Autodesk Inventor part; units mm, degrees
(part 2 of 3)
  line L955 (9.481, 12.2224) -> (9.3887, 12.173)
  line L956 (9.3887, 12.173) -> (9.2008, 12.0779)
  line L957 (9.2008, 12.0779) -> (8.8135, 11.9014)
  line L958 (8.8135, 11.9014) -> (8.4127, 11.7415)
  line L959 (8.4127, 11.7415) -> (7.9999, 11.5967)
  line L960 (7.9999, 11.5967) -> (7.5762, 11.4663)
  line L961 (7.5762, 11.4663) -> (7.1423, 11.3497)
  line L962 (7.1423, 11.3497) -> (6.777, 11.8009)
  line L963 (6.777, 11.8009) -> (6.9813, 12.201)
  line L964 (6.9813, 12.201) -> (7.1969, 12.5884)
  line L965 (7.1969, 12.5884) -> (7.4243, 12.9621)
  line L966 (7.4243, 12.9621) -> (7.6641, 13.3208)
  line L967 (7.6641, 13.3208) -> (7.9172, 13.663)
  line L968 (7.9172, 13.663) -> (8.0493, 13.827)
  line L969 (8.0493, 13.827) -> (8.1169, 13.907)
  line L970 (8.1169, 13.907) -> (8.1855, 13.9856)
  line L971 (8.1855, 13.9856) -> (7.7098, 14.6404)
  line L972 (7.7098, 14.6404) -> (7.6138, 14.5994)
  line L973 (7.6138, 14.5994) -> (7.5168, 14.5599)
  line L974 (7.5168, 14.5599) -> (7.32, 14.4849)
  line L975 (7.32, 14.4849) -> (6.9164, 14.3499)
  line L976 (6.9164, 14.3499) -> (6.5011, 14.2327)
  line L977 (6.5011, 14.2327) -> (6.0755, 14.1319)
  line L978 (6.0755, 14.1319) -> (5.6404, 14.0465)
  line L979 (5.6404, 14.0465) -> (5.1967, 13.9759)
  line L980 (5.1967, 13.9759) -> (4.8805, 14.4628)
  line L981 (4.8805, 14.4628) -> (5.1255, 14.8394)
  line L982 (5.1255, 14.8394) -> (5.3805, 15.2021)
  line L983 (5.3805, 15.2021) -> (5.6457, 15.55)
  line L984 (5.6457, 15.55) -> (5.9217, 15.8817)
  line L985 (5.9217, 15.8817) -> (6.2092, 16.1955)
  line L986 (6.2092, 16.1955) -> (6.3577, 16.3448)
  line L987 (6.3577, 16.3448) -> (6.4333, 16.4173)
  line L988 (6.4333, 16.4173) -> (6.5097, 16.4883)
  line L989 (6.5097, 16.4883) -> (6.1051, 17.1892)
  line L990 (6.1051, 17.1892) -> (6.0053, 17.1585)
  line L991 (6.0053, 17.1585) -> (5.9047, 17.1293)
  line L992 (5.9047, 17.1293) -> (5.7012, 17.0754)
  line L993 (5.7012, 17.0754) -> (5.2857, 16.9833)
  line L994 (5.2857, 16.9833) -> (4.8604, 16.9101)
  line L995 (4.8604, 16.9101) -> (4.4265, 16.8544)
  line L996 (4.4265, 16.8544) -> (3.9849, 16.8149)
  line L997 (3.9849, 16.8149) -> (3.5363, 16.7911)
  line L998 (3.5363, 16.7911) -> (3.2727, 17.3084)
  line L999 (3.2727, 17.3084) -> (3.5558, 17.6573)
  line L1000 (3.5558, 17.6573) -> (3.8472, 17.9913)
  line L1001 (3.8472, 17.9913) -> (4.1474, 18.3096)
  line L1002 (4.1474, 18.3096) -> (4.4565, 18.6106)
  line L1003 (4.4565, 18.6106) -> (4.7752, 18.8927)
  line L1004 (4.7752, 18.8927) -> (4.9385, 19.0256)
  line L1005 (4.9385, 19.0256) -> (5.0212, 19.0899)
  line L1006 (5.0212, 19.0899) -> (5.1047, 19.1525)
  line L1007 (5.1047, 19.1525) -> (4.7756, 19.8919)
  line L1008 (4.7756, 19.8919) -> (4.6731, 19.8717)
  line L1009 (4.6731, 19.8717) -> (4.5701, 19.8532)
  line L1010 (4.5701, 19.8532) -> (4.362, 19.8208)
  line L1011 (4.362, 19.8208) -> (3.9391, 19.7727)
  line L1012 (3.9391, 19.7727) -> (3.5085, 19.7444)
  line L1013 (3.5085, 19.7444) -> (3.0712, 19.7343)
  line L1014 (3.0712, 19.7343) -> (2.6279, 19.7412)
  line L1015 (2.6279, 19.7412) -> (2.1792, 19.7644)
  line L1016 (2.1792, 19.7644) -> (1.9712, 20.3064)
  line L1017 (1.9712, 20.3064) -> (2.2891, 20.6238)
  line L1018 (2.2891, 20.6238) -> (2.6139, 20.9256)
  line L1019 (2.6139, 20.9256) -> (2.9457, 21.2107)
  line L1020 (2.9457, 21.2107) -> (3.2846, 21.4778)
  line L1021 (3.2846, 21.4778) -> (3.631, 21.725)
  line L1022 (3.631, 21.725) -> (3.8074, 21.8401)
  line L1023 (3.8074, 21.8401) -> (3.8963, 21.8954)
  line L1024 (3.8963, 21.8954) -> (3.9859, 21.949)
  line L1025 (3.9859, 21.949) -> (3.7358, 22.7186)
  line L1026 (3.7358, 22.7186) -> (3.6319, 22.7093)
  line L1027 (3.6319, 22.7093) -> (3.5274, 22.7017)
  line L1028 (3.5274, 22.7017) -> (3.3171, 22.6913)
  line L1029 (3.3171, 22.6913) -> (2.8915, 22.6876)
  line L1030 (2.8915, 22.6876) -> (2.4603, 22.7045)
  line L1031 (2.4603, 22.7045) -> (2.0243, 22.7401)
  line L1032 (2.0243, 22.7401) -> (1.5842, 22.7933)
  line L1033 (1.5842, 22.7933) -> (1.1404, 22.8633)
  line L1034 (1.1404, 22.8633) -> (0.9901, 23.4241)
  line L1035 (0.9901, 23.4241) -> (1.3395, 23.7065)
  line L1036 (1.3395, 23.7065) -> (1.6941, 23.9727)
  line L1037 (1.6941, 23.9727) -> (2.0538, 24.2216)
  line L1038 (2.0538, 24.2216) -> (2.4188, 24.4518)
  line L1039 (2.4188, 24.4518) -> (2.7892, 24.6613)
  line L1040 (2.7892, 24.6613) -> (2.9766, 24.7575)
  line L1041 (2.9766, 24.7575) -> (3.0708, 24.8031)
  line L1042 (3.0708, 24.8031) -> (3.1655, 24.847)
  line L1043 (3.1655, 24.847) -> (2.9973, 25.6386)
  line L1044 (2.9973, 25.6386) -> (2.8929, 25.6402)
  line L1045 (2.8929, 25.6402) -> (2.7882, 25.6436)
  line L1046 (2.7882, 25.6436) -> (2.5779, 25.6552)
  line L1047 (2.5779, 25.6552) -> (2.1543, 25.696)
  line L1048 (2.1543, 25.696) -> (1.7273, 25.7578)
  line L1049 (1.7273, 25.7578) -> (1.2974, 25.8389)
  line L1050 (1.2974, 25.8389) -> (0.8652, 25.9378)
  line L1051 (0.8652, 25.9378) -> (0.4312, 26.0538)
  line L1052 (0.4312, 26.0538) -> (0.3404, 26.6272)
  line L1053 (0.3404, 26.6272) -> (0.7173, 26.8716)
  line L1054 (0.7173, 26.8716) -> (1.0978, 27.0992)
  line L1055 (1.0978, 27.0992) -> (1.4816, 27.3091)
  line L1056 (1.4816, 27.3091) -> (1.8686, 27.4999)
  line L1057 (1.8686, 27.4999) -> (2.2589, 27.6697)
  line L1058 (2.2589, 27.6697) -> (2.4553, 27.7456)
  line L1059 (2.4553, 27.7456) -> (2.5538, 27.7812)
  line L1060 (2.5538, 27.7812) -> (2.6526, 27.8149)
  line L1061 (2.6526, 27.8149) -> (2.568, 28.6198)
  line L1062 (2.568, 28.6198) -> (2.4644, 28.6323)
  line L1063 (2.4644, 28.6323) -> (2.3606, 28.6466)
  line L1064 (2.3606, 28.6466) -> (2.1527, 28.6801)
  line L1065 (2.1527, 28.6801) -> (1.7356, 28.765)
  line L1066 (1.7356, 28.765) -> (1.3174, 28.8711)
  line L1067 (1.3174, 28.8711) -> (0.8983, 28.9967)
  line L1068 (0.8983, 28.9967) -> (0.4789, 29.1403)
  line L1069 (0.4789, 29.1403) -> (0.0593, 29.3009)
  line L1070 (0.0593, 29.3009) -> (0.029, 29.8807)
  line L1071 (0.029, 29.8807) -> (0.4294, 30.0843)
  line L1072 (0.4294, 30.0843) -> (0.8316, 30.2709)
  line L1073 (0.8316, 30.2709) -> (1.2352, 30.4396)
  line L1074 (1.2352, 30.4396) -> (1.64, 30.5889)
  line L1075 (1.64, 30.5889) -> (2.0459, 30.7169)
  line L1076 (2.0459, 30.7169) -> (2.2492, 30.772)
  line L1077 (2.2492, 30.772) -> (2.3509, 30.797)
  line L1078 (2.3509, 30.797) -> (2.4527, 30.8203)
  line L1079 (2.4527, 30.8203) -> (2.4527, 31.6296)
  circle A0 centre (31.2249, 31.2249) radius 0.5
  line L1080 (62.4057, 32.859) -> (0.0441, 29.5908) construction
derived "Base_part.ipt"
derived "gear_central_part_30.ipt"
sketch "Sketch9" plane through (0, 0, 0) normal (0, 1, 0) x (-1, 0, 0)
  circle A0 centre (0, 0) radius 15
  arc A1 (4.5, -13.2571) -> (5.5, -12.8744) centre (0, 0) ccw
  line L0 (0, 0) -> (20.2233, 0) construction
  line L1 (0, 0) -> (0, -27.3647) construction
  line L2 (0.2121, 2.4395) -> (2.4395, 0.2121)
  line L3 (2.4395, -0.2121) -> (0.2121, -2.4395)
  line L4 (-0.2121, -2.4395) -> (-2.4395, -0.2121)
  line L5 (-2.4395, 0.2121) -> (-0.2121, 2.4395)
  line L6 (0, 2.6517) -> (0, -2.6517) construction
  line L7 (2.6517, 0) -> (-2.6517, 0) construction
  arc A2 (2.4395, -0.2121) -> (2.4395, 0.2121) centre (2.2274, 0) ccw
  arc A3 (-0.2121, -2.4395) -> (0.2121, -2.4395) centre (0, -2.2274) ccw
  arc A4 (-2.4395, 0.2121) -> (-2.4395, -0.2121) centre (-2.2274, 0) ccw
  arc A5 (0.2121, 2.4395) -> (-0.2121, 2.4395) centre (0, 2.2274) ccw
  line L8 (-3.1466, -0.9192) -> (-0.9192, -3.1466)
  arc A6 (-0.9192, -3.1466) -> (0.9192, -3.1466) centre (0, -2.2274) ccw
  line L9 (0.9192, -3.1466) -> (3.1466, -0.9192)
  arc A7 (3.1466, -0.9192) -> (3.1466, 0.9192) centre (2.2274, 0) ccw
  line L10 (3.1466, 0.9192) -> (0.9192, 3.1466)
  arc A8 (0.9192, 3.1466) -> (-0.9192, 3.1466) centre (0, 2.2274) ccw
  line L11 (-0.9192, 3.1466) -> (-3.1466, 0.9192)
  arc A9 (-3.1466, 0.9192) -> (-3.1466, -0.9192) centre (-2.2274, 0) ccw
  circle A10 centre (10, 0) radius 2.5
  arc A11 (13.4641, -0.5) -> (9.5, -3.4641) centre (10, 0) ccw
  line L12 (3.4274, -0.5) -> (6.5359, -0.5)
  line L13 (3.4274, 0.5) -> (6.5359, 0.5)
  line L14 (13.9911, 0.5) -> (13.4641, 0.5)
  line L15 (13.9911, -0.5) -> (13.4641, -0.5)
  line L16 (0, -5) -> (13.0767, -5) construction
  line L17 (0, -4.5) -> (13.2571, -4.5)
  line L18 (0, -5.5) -> (12.8744, -5.5)
  line L19 (5, 0) -> (5, -13.0767) construction
  line L20 (5.5, 12.8744) -> (5.5, -12.8744)
  line L21 (4.5, 13.2571) -> (4.5, -13.2571)
  arc A12 (0, -14) -> (4.5, -13.2571) centre (0, 0) ccw
  arc A13 (5.5, -12.8744) -> (12.8744, -5.5) centre (0, 0) ccw
  arc A14 (12.8744, -5.5) -> (13.2571, -4.5) centre (0, 0) ccw
  arc A15 (13.2571, -4.5) -> (13.9911, -0.5) centre (0, 0) ccw
  arc A16 (13.9911, -0.5) -> (13.9911, 0.5) centre (0, 0) ccw
  arc A17 (13.9911, 0.5) -> (5.5, 12.8744) centre (0, 0) ccw
  line L22 (0.5, -4.5) -> (0.5, -5.5)
  line L23 (10, 0) -> (10, -4.5) construction
  line L24 (10.5, -3.4641) -> (10.5, -4.5)
  line L25 (9.5, -3.4641) -> (9.5, -4.5)
  arc A18 (10.5, -3.4641) -> (13.4641, -0.5) centre (10, 0) ccw
  arc A19 (9.5, -3.4641) -> (10.5, -3.4641) centre (10, 0) ccw
  arc A20 (10.5, 3.4641) -> (9.5, 3.4641) centre (10, 0) ccw
  line L26 (0, -4.5) -> (0, -5.5)
  arc A21 (4.5, 13.2571) -> (0, -14) centre (0, 0) ccw
  arc A22 (5.5, 12.8744) -> (4.5, 13.2571) centre (0, 0) ccw
  line L27 (0, 4.5) -> (0, 5.5)
  line L28 (9.5, 3.4641) -> (9.5, 4.5)
  arc A23 (10.5, 3.4641) -> (9.5, 3.4641) centre (10, 0) ccw
  line L29 (0.5, 4.5) -> (0.5, 5.5)
  line L30 (0, 4.5) -> (13.2571, 4.5)
  line L31 (0, 5) -> (13.0767, 5) construction
  line L32 (0, 5.5) -> (12.8744, 5.5)
  arc A24 (13.2571, 4.5) -> (12.8744, 5.5) centre (0, 0) ccw
  line L33 (10.5, 3.4641) -> (10.5, 4.5)
  arc A25 (2.4395, -0.2121) -> (2.4395, 0.2121) centre (2.2274, 0) ccw
  line L34 (0.2121, 2.4395) -> (2.4395, 0.2121)
  line L35 (0.9192, -3.1466) -> (3.1466, -0.9192)
  arc A26 (0.2121, 2.4395) -> (-0.2121, 2.4395) centre (0, 2.2274) ccw
  line L36 (2.4395, -0.2121) -> (0.2121, -2.4395)
  line L37 (0, 2.6517) -> (0, -2.6517) construction
  line L38 (-2.4395, 0.2121) -> (-0.2121, 2.4395)
  line L39 (-2.6517, 0) -> (2.6517, 0) construction
  arc A27 (-0.2121, -2.4395) -> (0.2121, -2.4395) centre (0, -2.2274) ccw
  line L40 (-0.2121, -2.4395) -> (-2.4395, -0.2121)
  arc A28 (3.1466, -0.9192) -> (3.1466, 0.9192) centre (2.2274, 0) ccw
  line L41 (3.1466, 0.9192) -> (0.9192, 3.1466)
  line L42 (4.5, 0.5) -> (5.5, 0.5)
  line L43 (4.5, 0) -> (5.5, 0)
  line L44 (-13.2571, 4.5) -> (13.2571, 4.5)
  line L45 (0, 5) -> (13.0767, 5) construction
  arc A29 (14, 0) -> (13.2571, 4.5) centre (0, 0) ccw
  arc A30 (-0.9192, -3.1466) -> (0.9192, -3.1466) centre (0, -2.2274) ccw
  line L46 (-3.1466, -0.9192) -> (-0.9192, -3.1466)
  arc A31 (-12.8744, 5.5) -> (-13.2571, 4.5) centre (0, 0) ccw
  circle A32 centre (0, 10) radius 2.5
  arc A33 (0.5, 13.4641) -> (3.4641, 9.5) centre (0, 10) ccw
  line L47 (0.5, 3.4274) -> (0.5, 6.5359)
  line L48 (-0.5, 3.4274) -> (-0.5, 6.5359)
  arc A34 (3.4641, 10.5) -> (0.5, 13.4641) centre (0, 10) ccw
  line L49 (0, 10) -> (4.5, 10) construction
  line L50 (0.5, 13.9911) -> (0.5, 13.4641)
  arc A35 (4.5, 13.2571) -> (0.5, 13.9911) centre (0, 0) ccw
  line L51 (-12.8744, 5.5) -> (12.8744, 5.5)
  arc A36 (0.5, 13.9911) -> (-0.5, 13.9911) centre (0, 0) ccw
  line L52 (-0.5, 13.9911) -> (-0.5, 13.4641)
  arc A37 (13.2571, 4.5) -> (12.8744, 5.5) centre (0, 0) ccw
  arc A38 (3.4641, 9.5) -> (3.4641, 10.5) centre (0, 10) ccw
  line L53 (3.4641, 9.5) -> (4.5, 9.5)
  line L54 (3.4641, 10.5) -> (4.5, 10.5)
  arc A39 (5.5, 12.8744) -> (4.5, 13.2571) centre (0, 0) ccw
  line L55 (4.5, 0) -> (4.5, 13.2571)
  line L56 (5, 0) -> (5, 13.0767) construction
  line L57 (5.5, 0) -> (5.5, 12.8744)
  arc A40 (12.8744, 5.5) -> (5.5, 12.8744) centre (0, 0) ccw
  line L58 (-0.9192, 3.1466) -> (-3.1466, 0.9192)
  arc A41 (-3.4641, 10.5) -> (-3.4641, 9.5) centre (0, 10) ccw
  arc A42 (-3.4641, 10.5) -> (-3.4641, 9.5) centre (0, 10) ccw
  line L59 (-3.4641, 10.5) -> (-4.5, 10.5)
  line L60 (-4.5, 0) -> (-4.5, 13.2571)
  line L61 (-5, 0) -> (-5, 13.0767) construction
  line L62 (-5.5, 0) -> (-5.5, 12.8744)
  arc A43 (-4.5, 13.2571) -> (-5.5, 12.8744) centre (0, 0) ccw
  arc A44 (-0.5, 13.9911) -> (-12.8744, 5.5) centre (0, 0) ccw
  line L63 (-3.4641, 9.5) -> (-4.5, 9.5)
  line L64 (-4.5, 0.5) -> (-5.5, 0.5)
  line L65 (-4.5, 0) -> (-5.5, 0)
  arc A45 (-2.4395, 0.2121) -> (-2.4395, -0.2121) centre (-2.2274, 0) ccw
  arc A46 (-3.1466, 0.9192) -> (-3.1466, -0.9192) centre (-2.2274, 0) ccw
  arc A47 (0.9192, 3.1466) -> (-0.9192, 3.1466) centre (0, 2.2274) ccw
  arc A48 (0.2121, 2.4395) -> (-0.2121, 2.4395) centre (0, 2.2274) ccw
  line L66 (-2.4395, 0.2121) -> (-0.2121, 2.4395)
  line L67 (3.1466, 0.9192) -> (0.9192, 3.1466)
  arc A49 (-2.4395, 0.2121) -> (-2.4395, -0.2121) centre (-2.2274, 0) ccw
  line L68 (0.2121, 2.4395) -> (2.4395, 0.2121)
  line L69 (-2.6517, 0) -> (2.6517, 0) construction
  line L70 (-0.2121, -2.4395) -> (-2.4395, -0.2121)
  line L71 (0, -2.6517) -> (0, 2.6517) construction
  arc A50 (2.4395, -0.2121) -> (2.4395, 0.2121) centre (2.2274, 0) ccw
  line L72 (2.4395, -0.2121) -> (0.2121, -2.4395)
  arc A51 (0.9192, 3.1466) -> (-0.9192, 3.1466) centre (0, 2.2274) ccw
  line L73 (-0.9192, 3.1466) -> (-3.1466, 0.9192)
  line L74 (-0.5, 4.5) -> (-0.5, 5.5)
  line L75 (0, 4.5) -> (0, 5.5)
  line L76 (-4.5, -13.2571) -> (-4.5, 13.2571)
  line L77 (-5, 0) -> (-5, 13.0767) construction
  arc A52 (0, 14) -> (-4.5, 13.2571) centre (0, 0) ccw
  arc A53 (3.1466, -0.9192) -> (3.1466, 0.9192) centre (2.2274, 0) ccw
  line L78 (0.9192, -3.1466) -> (3.1466, -0.9192)
  arc A54 (-5.5, -12.8744) -> (-4.5, -13.2571) centre (0, 0) ccw
  circle A55 centre (-10, 0) radius 2.5
  arc A56 (-13.4641, 0.5) -> (-9.5, 3.4641) centre (-10, 0) ccw
  line L79 (-3.4274, 0.5) -> (-6.5359, 0.5)
  line L80 (-3.4274, -0.5) -> (-6.5359, -0.5)
  arc A57 (-10.5, 3.4641) -> (-13.4641, 0.5) centre (-10, 0) ccw
  line L81 (-10, 0) -> (-10, 4.5) construction
  line L82 (-13.9911, 0.5) -> (-13.4641, 0.5)
  arc A58 (-13.2571, 4.5) -> (-13.9911, 0.5) centre (0, 0) ccw
  line L83 (-5.5, -12.8744) -> (-5.5, 12.8744)
  arc A59 (-13.9911, 0.5) -> (-13.9911, -0.5) centre (0, 0) ccw
  line L84 (-13.9911, -0.5) -> (-13.4641, -0.5)
  arc A60 (-4.5, 13.2571) -> (-5.5, 12.8744) centre (0, 0) ccw
  arc A61 (-9.5, 3.4641) -> (-10.5, 3.4641) centre (-10, 0) ccw
  line L85 (-9.5, 3.4641) -> (-9.5, 4.5)
  line L86 (-10.5, 3.4641) -> (-10.5, 4.5)
  arc A62 (-12.8744, 5.5) -> (-13.2571, 4.5) centre (0, 0) ccw
  line L87 (0, 4.5) -> (-13.2571, 4.5)
  line L88 (0, 5) -> (-13.0767, 5) construction
  line L89 (0, 5.5) -> (-12.8744, 5.5)
  arc A63 (-5.5, 12.8744) -> (-12.8744, 5.5) centre (0, 0) ccw
  line L90 (-3.1466, -0.9192) -> (-0.9192, -3.1466)
  arc A64 (-10.5, -3.4641) -> (-9.5, -3.4641) centre (-10, 0) ccw
  arc A65 (-10.5, -3.4641) -> (-9.5, -3.4641) centre (-10, 0) ccw
  line L91 (-10.5, -3.4641) -> (-10.5, -4.5)
  line L92 (0, -4.5) -> (-13.2571, -4.5)
  line L93 (0, -5) -> (-13.0767, -5) construction
  line L94 (0, -5.5) -> (-12.8744, -5.5)
  arc A66 (-13.2571, -4.5) -> (-12.8744, -5.5) centre (0, 0) ccw
  arc A67 (-13.9911, -0.5) -> (-5.5, -12.8744) centre (0, 0) ccw
  line L95 (-9.5, -3.4641) -> (-9.5, -4.5)
  line L96 (-0.5, -4.5) -> (-0.5, -5.5)
  line L97 (0, -4.5) -> (0, -5.5)
  arc A68 (-0.2121, -2.4395) -> (0.2121, -2.4395) centre (0, -2.2274) ccw
  arc A69 (-0.9192, -3.1466) -> (0.9192, -3.1466) centre (0, -2.2274) ccw
  arc A70 (-3.1466, 0.9192) -> (-3.1466, -0.9192) centre (-2.2274, 0) ccw
  arc A71 (-2.4395, 0.2121) -> (-2.4395, -0.2121) centre (-2.2274, 0) ccw
  line L98 (-0.2121, -2.4395) -> (-2.4395, -0.2121)
  line L99 (-0.9192, 3.1466) -> (-3.1466, 0.9192)
  arc A72 (-0.2121, -2.4395) -> (0.2121, -2.4395) centre (0, -2.2274) ccw
  line L100 (-2.4395, 0.2121) -> (-0.2121, 2.4395)
  line L101 (0, -2.6517) -> (0, 2.6517) construction
  line L102 (2.4395, -0.2121) -> (0.2121, -2.4395)
  line L103 (2.6517, 0) -> (-2.6517, 0) construction
  arc A73 (0.2121, 2.4395) -> (-0.2121, 2.4395) centre (0, 2.2274) ccw
  line L104 (0.2121, 2.4395) -> (2.4395, 0.2121)
  arc A74 (-3.1466, 0.9192) -> (-3.1466, -0.9192) centre (-2.2274, 0) ccw
  line L105 (-3.1466, -0.9192) -> (-0.9192, -3.1466)
  line L106 (-4.5, -0.5) -> (-5.5, -0.5)
  line L107 (-4.5, 0) -> (-5.5, 0)
  line L108 (13.2571, -4.5) -> (-13.2571, -4.5)
  line L109 (0, -5) -> (-13.0767, -5) construction
  arc A75 (-14, 0) -> (-13.2571, -4.5) centre (0, 0) ccw
  arc A76 (0.9192, 3.1466) -> (-0.9192, 3.1466) centre (0, 2.2274) ccw
  line L110 (3.1466, 0.9192) -> (0.9192, 3.1466)
  arc A77 (12.8744, -5.5) -> (13.2571, -4.5) centre (0, 0) ccw
  circle A78 centre (0, -10) radius 2.5
  arc A79 (-0.5, -13.4641) -> (-3.4641, -9.5) centre (0, -10) ccw
  line L111 (-0.5, -3.4274) -> (-0.5, -6.5359)
  line L112 (0.5, -3.4274) -> (0.5, -6.5359)
  arc A80 (-3.4641, -10.5) -> (-0.5, -13.4641) centre (0, -10) ccw
  line L113 (0, -10) -> (-4.5, -10) construction
  line L114 (-0.5, -13.9911) -> (-0.5, -13.4641)
  arc A81 (-4.5, -13.2571) -> (-0.5, -13.9911) centre (0, 0) ccw
  line L115 (12.8744, -5.5) -> (-12.8744, -5.5)
  arc A82 (-0.5, -13.9911) -> (0.5, -13.9911) centre (0, 0) ccw
  line L116 (0.5, -13.9911) -> (0.5, -13.4641)
  arc A83 (-13.2571, -4.5) -> (-12.8744, -5.5) centre (0, 0) ccw
  arc A84 (-3.4641, -9.5) -> (-3.4641, -10.5) centre (0, -10) ccw
  line L117 (-3.4641, -9.5) -> (-4.5, -9.5)
  line L118 (-3.4641, -10.5) -> (-4.5, -10.5)
  arc A85 (-5.5, -12.8744) -> (-4.5, -13.2571) centre (0, 0) ccw
  line L119 (-4.5, 0) -> (-4.5, -13.2571)
  line L120 (-5, 0) -> (-5, -13.0767) construction
  line L121 (-5.5, 0) -> (-5.5, -12.8744)
  arc A86 (-12.8744, -5.5) -> (-5.5, -12.8744) centre (0, 0) ccw
  line L122 (0.9192, -3.1466) -> (3.1466, -0.9192)
  arc A87 (3.4641, -10.5) -> (3.4641, -9.5) centre (0, -10) ccw
  arc A88 (3.4641, -10.5) -> (3.4641, -9.5) centre (0, -10) ccw
  line L123 (3.4641, -10.5) -> (4.5, -10.5)
  line L124 (4.5, 0) -> (4.5, -13.2571)
  line L125 (5, 0) -> (5, -13.0767) construction
  line L126 (5.5, 0) -> (5.5, -12.8744)
  arc A89 (4.5, -13.2571) -> (5.5, -12.8744) centre (0, 0) ccw
  arc A90 (0.5, -13.9911) -> (12.8744, -5.5) centre (0, 0) ccw
  line L127 (3.4641, -9.5) -> (4.5, -9.5)
  line L128 (4.5, -0.5) -> (5.5, -0.5)
  line L129 (4.5, 0) -> (5.5, 0)
  arc A91 (2.4395, -0.2121) -> (2.4395, 0.2121) centre (2.2274, 0) ccw
  arc A92 (3.1466, -0.9192) -> (3.1466, 0.9192) centre (2.2274, 0) ccw
  arc A93 (-0.9192, -3.1466) -> (0.9192, -3.1466) centre (0, -2.2274) ccw
  point P0 (0, 2.2274)
  point P1 (10, 4.5)
  point P2 (-4.5, 10)
  point P3 (-2.2274, 0)
  point P4 (-10, -4.5)
  point P5 (0, -2.2274)
  point P6 (4.5, -10)
  point P7 (2.2274, 0)
sketch "Sketch7" plane through (0, 0, 0) normal (0, 1, 0) x (-1, 0, 0)
  line L0 (0.8173, 31.2129) -> (-0.8173, -31.2129) construction
  arc A0 (4.5, 27.4052) -> (-4.5, 27.4052) centre (0, 0) ccw
  line L1 (5.5, 13.9553) -> (5.5, 27.2222)
  line L2 (4.5, 14.3091) -> (4.5, 27.4052)
  line L3 (5.5, 0) -> (5.5, 12.8744) projected
  line L4 (4.5, 0) -> (4.5, 13.2571) projected
  line L5 (-4.5, 0) -> (-4.5, 13.2571) projected
  line L6 (-5.5, -12.8744) -> (-5.5, 12.8744) projected
  circle A1 centre (0, 0) radius 15 projected
  line L7 (-4.5, 14.3091) -> (-4.5, 27.4052)
  line L8 (-5.5, 13.9553) -> (-5.5, 27.2222)
  arc A2 (5.5, 27.2222) -> (4.5, 27.4052) centre (0, 0) ccw
  arc A3 (-5.5, 27.2222) -> (5.5, 27.2222) centre (0, 0) ccw
  arc A4 (-4.5, 27.4052) -> (-5.5, 27.2222) centre (0, 0) ccw
  arc A5 (5.5, 13.9553) -> (4.5, 14.3091) centre (0, 0) ccw
  arc A6 (-4.5, 14.3091) -> (-5.5, 13.9553) centre (0, 0) ccw
  arc A7 (-14.3091, -4.5) -> (-13.9553, -5.5) centre (0, 0) ccw
  arc A8 (-13.9553, 5.5) -> (-14.3091, 4.5) centre (0, 0) ccw
  line L9 (-13.9553, 5.5) -> (-27.2222, 5.5)
  line L10 (-14.3091, 4.5) -> (-27.4052, 4.5)
  arc A9 (-27.2222, 5.5) -> (-27.4052, 4.5) centre (0, 0) ccw
  line L11 (-14.3091, -4.5) -> (-27.4052, -4.5)
  line L12 (-13.9553, -5.5) -> (-27.2222, -5.5)
  arc A10 (-27.4052, -4.5) -> (-27.2222, -5.5) centre (0, 0) ccw
  arc A11 (4.5, -14.3091) -> (5.5, -13.9553) centre (0, 0) ccw
  arc A12 (-5.5, -13.9553) -> (-4.5, -14.3091) centre (0, 0) ccw
  line L13 (-5.5, -13.9553) -> (-5.5, -27.2222)
  line L14 (-4.5, -14.3091) -> (-4.5, -27.4052)
  arc A13 (-5.5, -27.2222) -> (-4.5, -27.4052) centre (0, 0) ccw
  line L15 (4.5, -14.3091) -> (4.5, -27.4052)
  line L16 (5.5, -13.9553) -> (5.5, -27.2222)
  arc A14 (4.5, -27.4052) -> (5.5, -27.2222) centre (0, 0) ccw
  arc A15 (14.3091, 4.5) -> (13.9553, 5.5) centre (0, 0) ccw
  arc A16 (13.9553, -5.5) -> (14.3091, -4.5) centre (0, 0) ccw
  line L17 (13.9553, -5.5) -> (27.2222, -5.5)
  line L18 (14.3091, -4.5) -> (27.4052, -4.5)
  arc A17 (27.2222, -5.5) -> (27.4052, -4.5) centre (0, 0) ccw
  line L19 (14.3091, 4.5) -> (27.4052, 4.5)
  line L20 (13.9553, 5.5) -> (27.2222, 5.5)
  arc A18 (27.4052, 4.5) -> (27.2222, 5.5) centre (0, 0) ccw
  arc A19 (14.7224, 8.5) -> (8.5, 14.7224) centre (0, 0) ccw
  line L21 (16.4545, 7.5) -> (21.7915, 7.5)
  line L22 (7.5, 16.4545) -> (7.5, 21.7915)
  arc A20 (23.6249, 10.2993) -> (10.2993, 23.6249) centre (0, 0) ccw
  arc A21 (21.7915, 7.5) -> (23.6249, 10.2993) centre (21.7915, 9.5) ccw
  arc A22 (14.7224, 8.5) -> (16.4545, 7.5) centre (16.4545, 9.5) ccw
  arc A23 (7.5, 16.4545) -> (8.5, 14.7224) centre (9.5, 16.4545) ccw
  arc A24 (10.2993, 23.6249) -> (7.5, 21.7915) centre (9.5, 21.7915) ccw
  arc A25 (-16.4545, 7.5) -> (-14.7224, 8.5) centre (-16.4545, 9.5) ccw
  line L23 (-16.4545, 7.5) -> (-21.7915, 7.5)
  arc A26 (-23.6249, 10.2993) -> (-21.7915, 7.5) centre (-21.7915, 9.5) ccw
  arc A27 (-8.5, 14.7224) -> (-14.7224, 8.5) centre (0, 0) ccw
  arc A28 (-10.2993, 23.6249) -> (-23.6249, 10.2993) centre (0, 0) ccw
  arc A29 (-8.5, 14.7224) -> (-7.5, 16.4545) centre (-9.5, 16.4545) ccw
  line L24 (-7.5, 16.4545) -> (-7.5, 21.7915)
  arc A30 (-7.5, 21.7915) -> (-10.2993, 23.6249) centre (-9.5, 21.7915) ccw
  arc A31 (-7.5, -16.4545) -> (-8.5, -14.7224) centre (-9.5, -16.4545) ccw
  line L25 (-7.5, -16.4545) -> (-7.5, -21.7915)
  arc A32 (-10.2993, -23.6249) -> (-7.5, -21.7915) centre (-9.5, -21.7915) ccw
  arc A33 (-14.7224, -8.5) -> (-8.5, -14.7224) centre (0, 0) ccw
  arc A34 (-23.6249, -10.2993) -> (-10.2993, -23.6249) centre (0, 0) ccw
  arc A35 (-14.7224, -8.5) -> (-16.4545, -7.5) centre (-16.4545, -9.5) ccw
  line L26 (-16.4545, -7.5) -> (-21.7915, -7.5)
  arc A36 (-21.7915, -7.5) -> (-23.6249, -10.2993) centre (-21.7915, -9.5) ccw
  arc A37 (16.4545, -7.5) -> (14.7224, -8.5) centre (16.4545, -9.5) ccw
  line L27 (16.4545, -7.5) -> (21.7915, -7.5)
  arc A38 (23.6249, -10.2993) -> (21.7915, -7.5) centre (21.7915, -9.5) ccw
  arc A39 (8.5, -14.7224) -> (14.7224, -8.5) centre (0, 0) ccw
  arc A40 (10.2993, -23.6249) -> (23.6249, -10.2993) centre (0, 0) ccw
  arc A41 (8.5, -14.7224) -> (7.5, -16.4545) centre (9.5, -16.4545) ccw
  line L28 (7.5, -16.4545) -> (7.5, -21.7915)
  arc A42 (7.5, -21.7915) -> (10.2993, -23.6249) centre (9.5, -21.7915) ccw
  line L29 (0, 0) -> (0, -11.3594) construction
  line L30 (-28.6518, 2.6609) -> (-28.7514, 2.692)
  line L31 (-28.7514, 2.692) -> (-28.8508, 2.725)
  line L32 (-28.8508, 2.725) -> (-29.0492, 2.7958)
  line L33 (-29.0492, 2.7958) -> (-29.4438, 2.9552)
  line L34 (-29.4438, 2.9552) -> (-29.8357, 3.1359)
  line L35 (-29.8357, 3.1359) -> (-30.2248, 3.3356)
  line L36 (-30.2248, 3.3356) -> (-30.6111, 3.5533)
  line L37 (-30.6111, 3.5533) -> (-30.9943, 3.7877)
  line L38 (-30.9943, 3.7877) -> (-30.9185, 4.3633)
  line L39 (-30.9185, 4.3633) -> (-30.4877, 4.4905)
  line L40 (-30.4877, 4.4905) -> (-30.0582, 4.6008)
  line L41 (-30.0582, 4.6008) -> (-29.6306, 4.693)
  line L42 (-29.6306, 4.693) -> (-29.2054, 4.7661)
  line L43 (-29.2054, 4.7661) -> (-28.7829, 4.8179)
  line L44 (-28.7829, 4.8179) -> (-28.573, 4.835)
  line L45 (-28.573, 4.835) -> (-28.4685, 4.8411)
  line L46 (-28.4685, 4.8411) -> (-28.3642, 4.8455)
  line L47 (-28.3642, 4.8455) -> (-28.2167, 5.6412)
  line L48 (-28.2167, 5.6412) -> (-28.3125, 5.6826)
  line L49 (-28.3125, 5.6826) -> (-28.408, 5.7258)
  line L50 (-28.408, 5.7258) -> (-28.5978, 5.817)
  line L51 (-28.5978, 5.817) -> (-28.9736, 6.0168)
  line L52 (-28.9736, 6.0168) -> (-29.3444, 6.2374)
  line L53 (-29.3444, 6.2374) -> (-29.7105, 6.4767)
  line L54 (-29.7105, 6.4767) -> (-30.072, 6.7335)
  line L55 (-30.072, 6.7335) -> (-30.4286, 7.0067)
  line L56 (-30.4286, 7.0067) -> (-30.2931, 7.5713)
  line L57 (-30.2931, 7.5713) -> (-29.8513, 7.6528)
  line L58 (-29.8513, 7.6528) -> (-29.4127, 7.7175)
  line L59 (-29.4127, 7.7175) -> (-28.9778, 7.7646)
  line L60 (-28.9778, 7.7646) -> (-28.5472, 7.7928)
  line L61 (-28.5472, 7.7928) -> (-28.1217, 7.8002)
  line L62 (-28.1217, 7.8002) -> (-27.9111, 7.7952)
  line L63 (-27.9111, 7.7952) -> (-27.8065, 7.7904)
  line L64 (-27.8065, 7.7904) -> (-27.7023, 7.7838)
  line L65 (-27.7023, 7.7838) -> (-27.4725, 8.5597)
  line L66 (-27.4725, 8.5597) -> (-27.5634, 8.611)
  line L67 (-27.5634, 8.611) -> (-27.6538, 8.6638)
  line L68 (-27.6538, 8.6638) -> (-27.8331, 8.7744)
  line L69 (-27.8331, 8.7744) -> (-28.1859, 9.0124)
  line L70 (-28.1859, 9.0124) -> (-28.5317, 9.2705)
  line L71 (-28.5317, 9.2705) -> (-28.8708, 9.5469)
  line L72 (-28.8708, 9.5469) -> (-29.2034, 9.84)
  line L73 (-29.2034, 9.84) -> (-29.5295, 10.149)
  line L74 (-29.5295, 10.149) -> (-29.3357, 10.6963)
  line L75 (-29.3357, 10.6963) -> (-28.8878, 10.7312)
  line L76 (-28.8878, 10.7312) -> (-28.4448, 10.7497)
  line L77 (-28.4448, 10.7497) -> (-28.0074, 10.751)
  line L78 (-28.0074, 10.751) -> (-27.5762, 10.7341)
  line L79 (-27.5762, 10.7341) -> (-27.1523, 10.697)
  line L80 (-27.1523, 10.697) -> (-26.9434, 10.67)
  line L81 (-26.9434, 10.67) -> (-26.8399, 10.6543)
  line L82 (-26.8399, 10.6543) -> (-26.7369, 10.6368)
  line L83 (-26.7369, 10.6368) -> (-26.4272, 11.3845)
  line L84 (-26.4272, 11.3845) -> (-26.5123, 11.4449)
  line L85 (-26.5123, 11.4449) -> (-26.5967, 11.507)
  line L86 (-26.5967, 11.507) -> (-26.7634, 11.6356)
  line L87 (-26.7634, 11.6356) -> (-27.0895, 11.9092)
  line L88 (-27.0895, 11.9092) -> (-27.4064, 12.2021)
  line L89 (-27.4064, 12.2021) -> (-27.7147, 12.5124)
  line L90 (-27.7147, 12.5124) -> (-28.0148, 12.8387)
  line L91 (-28.0148, 12.8387) -> (-28.3069, 13.1801)
  line L92 (-28.3069, 13.1801) -> (-28.0569, 13.7041)
  line L93 (-28.0569, 13.7041) -> (-27.6078, 13.692)
  line L94 (-27.6078, 13.692) -> (-27.1654, 13.6641)
  line L95 (-27.1654, 13.6641) -> (-26.7302, 13.6197)
  line L96 (-26.7302, 13.6197) -> (-26.3032, 13.5578)
  line L97 (-26.3032, 13.5578) -> (-25.8854, 13.4766)
  line L98 (-25.8854, 13.4766) -> (-25.6805, 13.4279)
  line L99 (-25.6805, 13.4279) -> (-25.5791, 13.4014)
  line L100 (-25.5791, 13.4014) -> (-25.4786, 13.3733)
  line L101 (-25.4786, 13.3733) -> (-25.0925, 14.0845)
  line L102 (-25.0925, 14.0845) -> (-25.1708, 14.1535)
  line L103 (-25.1708, 14.1535) -> (-25.2482, 14.2241)
  line L104 (-25.2482, 14.2241) -> (-25.4006, 14.3695)
  line L105 (-25.4006, 14.3695) -> (-25.6962, 14.6756)
  line L106 (-25.6962, 14.6756) -> (-25.9808, 15)
  line L107 (-25.9808, 15) -> (-26.255, 15.3408)
  line L108 (-26.255, 15.3408) -> (-26.5194, 15.6967)
  line L109 (-26.5194, 15.6967) -> (-26.7741, 16.0667)
  line L110 (-26.7741, 16.0667) -> (-26.4708, 16.5618)
  line L111 (-26.4708, 16.5618) -> (-26.0254, 16.5028)
  line L112 (-26.0254, 16.5028) -> (-25.5883, 16.4288)
  line L113 (-25.5883, 16.4288) -> (-25.1601, 16.3392)
  line L114 (-25.1601, 16.3392) -> (-24.7419, 16.2329)
  line L115 (-24.7419, 16.2329) -> (-24.3349, 16.1085)
  line L116 (-24.3349, 16.1085) -> (-24.1362, 16.0387)
  line L117 (-24.1362, 16.0387) -> (-24.0382, 16.0018)
  line L118 (-24.0382, 16.0018) -> (-23.9412, 15.9633)
  line L119 (-23.9412, 15.9633) -> (-23.4828, 16.6303)
  line L120 (-23.4828, 16.6303) -> (-23.5534, 16.7071)
  line L121 (-23.5534, 16.7071) -> (-23.6231, 16.7853)
  line L122 (-23.6231, 16.7853) -> (-23.7594, 16.9458)
  line L123 (-23.7594, 16.9458) -> (-24.0214, 17.2812)
  line L124 (-24.0214, 17.2812) -> (-24.2705, 17.6336)
  line L125 (-24.2705, 17.6336) -> (-24.5076, 18.0012)
  line L126 (-24.5076, 18.0012) -> (-24.7333, 18.3827)
  line L127 (-24.7333, 18.3827) -> (-24.948, 18.7774)
  line L128 (-24.948, 18.7774) -> (-24.5946, 19.238)
  line L129 (-24.5946, 19.238) -> (-24.1578, 19.1328)
  line L130 (-24.1578, 19.1328) -> (-23.7308, 19.0135)
  line L131 (-23.7308, 19.0135) -> (-23.3144, 18.8796)
  line L132 (-23.3144, 18.8796) -> (-22.9096, 18.7302)
  line L133 (-22.9096, 18.7302) -> (-22.5178, 18.5639)
  line L134 (-22.5178, 18.5639) -> (-22.3275, 18.4738)
  line L135 (-22.3275, 18.4738) -> (-22.2339, 18.4268)
  line L136 (-22.2339, 18.4268) -> (-22.1414, 18.3784)
  line L137 (-22.1414, 18.3784) -> (-21.6158, 18.9938)
  line L138 (-21.6158, 18.9938) -> (-21.6781, 19.0776)
  line L139 (-21.6781, 19.0776) -> (-21.7391, 19.1626)
  line L140 (-21.7391, 19.1626) -> (-21.8579, 19.3365)
  line L141 (-21.8579, 19.3365) -> (-22.0835, 19.6974)
  line L142 (-22.0835, 19.6974) -> (-22.2943, 20.0739)
  line L143 (-22.2943, 20.0739) -> (-22.4917, 20.4643)
  line L144 (-22.4917, 20.4643) -> (-22.6763, 20.8674)
  line L145 (-22.6763, 20.8674) -> (-22.8486, 21.2823)
  line L146 (-22.8486, 21.2823) -> (-22.4489, 21.7035)
  line L147 (-22.4489, 21.7035) -> (-22.0256, 21.5531)
  line L148 (-22.0256, 21.5531) -> (-21.6134, 21.3899)
  line L149 (-21.6134, 21.3899) -> (-21.2132, 21.2132)
  line L150 (-21.2132, 21.2132) -> (-20.8262, 21.0223)
  line L151 (-20.8262, 21.0223) -> (-20.454, 20.816)
  line L152 (-20.454, 20.816) -> (-20.2741, 20.7064)
  line L153 (-20.2741, 20.7064) -> (-20.1859, 20.6499)
  line L154 (-20.1859, 20.6499) -> (-20.099, 20.5921)
  line L155 (-20.099, 20.5921) -> (-19.512, 21.1492)
  line L156 (-19.512, 21.1492) -> (-19.5652, 21.239)
  line L157 (-19.5652, 21.239) -> (-19.617, 21.33)
  line L158 (-19.617, 21.33) -> (-19.717, 21.5154)
  line L159 (-19.717, 21.5154) -> (-19.9035, 21.8979)
  line L160 (-19.9035, 21.8979) -> (-20.0739, 22.2943)
  line L161 (-20.0739, 22.2943) -> (-20.2294, 22.7032)
  line L162 (-20.2294, 22.7032) -> (-20.3709, 23.1234)
  line L163 (-20.3709, 23.1234) -> (-20.4988, 23.5541)
  line L164 (-20.4988, 23.5541) -> (-20.0573, 23.9311)
  line L165 (-20.0573, 23.9311) -> (-19.652, 23.7374)
  line L166 (-19.652, 23.7374) -> (-19.2591, 23.5319)
  line L167 (-19.2591, 23.5319) -> (-18.8796, 23.3144)
  line L168 (-18.8796, 23.3144) -> (-18.5147, 23.0841)
  line L169 (-18.5147, 23.0841) -> (-18.1661, 22.84)
  line L170 (-18.1661, 22.84) -> (-17.9987, 22.7122)
  line L171 (-17.9987, 22.7122) -> (-17.9169, 22.6468)
  line L172 (-17.9169, 22.6468) -> (-17.8365, 22.5802)
  line L173 (-17.8365, 22.5802) -> (-17.1944, 23.0729)
  line L174 (-17.1944, 23.0729) -> (-17.2379, 23.1678)
  line L175 (-17.2379, 23.1678) -> (-17.2799, 23.2637)
  line L176 (-17.2799, 23.2637) -> (-17.36, 23.4585)
  line L177 (-17.36, 23.4585) -> (-17.5056, 23.8584)
  line L178 (-17.5056, 23.8584) -> (-17.6336, 24.2705)
  line L179 (-17.6336, 24.2705) -> (-17.7455, 24.6934)
  line L180 (-17.7455, 24.6934) -> (-17.8422, 25.1261)
  line L181 (-17.8422, 25.1261) -> (-17.9245, 25.5677)
  line L182 (-17.9245, 25.5677) -> (-17.446, 25.8966)
  line L183 (-17.446, 25.8966) -> (-17.0631, 25.6615)
  line L184 (-17.0631, 25.6615) -> (-16.6939, 25.4161)
  line L185 (-16.6939, 25.4161) -> (-16.3392, 25.1601)
  line L186 (-16.3392, 25.1601) -> (-16.0003, 24.8929)
  line L187 (-16.0003, 24.8929) -> (-15.6791, 24.6137)
  line L188 (-15.6791, 24.6137) -> (-15.526, 24.4692)
  line L189 (-15.526, 24.4692) -> (-15.4515, 24.3955)
  line L190 (-15.4515, 24.3955) -> (-15.3785, 24.3209)
  line L191 (-15.3785, 24.3209) -> (-14.6884, 24.7438)
  line L192 (-14.6884, 24.7438) -> (-14.7218, 24.8427)
  line L193 (-14.7218, 24.8427) -> (-14.7535, 24.9425)
  line L194 (-14.7535, 24.9425) -> (-14.8128, 25.1446)
  line L195 (-14.8128, 25.1446) -> (-14.9158, 25.5575)
  line L196 (-14.9158, 25.5575) -> (-15, 25.9808)
  line L197 (-15, 25.9808) -> (-15.0671, 26.413)
  line L198 (-15.0671, 26.413) -> (-15.1181, 26.8534)
  line L199 (-15.1181, 26.8534) -> (-15.1537, 27.3013)
  line L200 (-15.1537, 27.3013) -> (-14.6435, 27.5783)
  line L201 (-14.6435, 27.5783) -> (-14.2873, 27.3045)
  line L202 (-14.2873, 27.3045) -> (-13.9457, 27.0219)
  line L203 (-13.9457, 27.0219) -> (-13.6197, 26.7302)
  line L204 (-13.6197, 26.7302) -> (-13.3106, 26.4291)
  line L205 (-13.3106, 26.4291) -> (-13.0204, 26.1178)
  line L206 (-13.0204, 26.1178) -> (-12.8832, 25.958)
  line L207 (-12.8832, 25.958) -> (-12.8168, 25.877)
  line L208 (-12.8168, 25.877) -> (-12.752, 25.7952)
  line L209 (-12.752, 25.7952) -> (-12.0215, 26.1436)
  line L210 (-12.0215, 26.1436) -> (-12.0444, 26.2455)
  line L211 (-12.0444, 26.2455) -> (-12.0655, 26.348)
  line L212 (-12.0655, 26.348) -> (-12.1033, 26.5552)
  line L213 (-12.1033, 26.5552) -> (-12.1626, 26.9767)
  line L214 (-12.1626, 26.9767) -> (-12.2021, 27.4064)
  line L215 (-12.2021, 27.4064) -> (-12.2236, 27.8433)
  line L216 (-12.2236, 27.8433) -> (-12.2283, 28.2866)
  line L217 (-12.2283, 28.2866) -> (-12.2169, 28.7357)
  line L218 (-12.2169, 28.7357) -> (-11.6805, 28.9579)
  line L219 (-11.6805, 28.9579) -> (-11.3549, 28.6484)
  line L220 (-11.3549, 28.6484) -> (-11.0447, 28.3316)
  line L221 (-11.0447, 28.3316) -> (-10.751, 28.0074)
  line L222 (-10.751, 28.0074) -> (-10.4751, 27.6756)
  line L223 (-10.4751, 27.6756) -> (-10.219, 27.3357)
  line L224 (-10.219, 27.3357) -> (-10.0993, 27.1625)
  line L225 (-10.0993, 27.1625) -> (-10.0417, 27.075)
  line L226 (-10.0417, 27.075) -> (-9.9858, 26.9868)
  line L227 (-9.9858, 26.9868) -> (-9.2229, 27.257)
  line L228 (-9.2229, 27.257) -> (-9.235, 27.3607)
  line L229 (-9.235, 27.3607) -> (-9.2453, 27.4649)
  line L230 (-9.2453, 27.4649) -> (-9.2613, 27.6749)
  line L231 (-9.2613, 27.6749) -> (-9.2761, 28.1002)
  line L232 (-9.2761, 28.1002) -> (-9.2705, 28.5317)
  line L233 (-9.2705, 28.5317) -> (-9.2463, 28.9685)
  line L234 (-9.2463, 28.9685) -> (-9.2046, 29.4098)
  line L235 (-9.2046, 29.4098) -> (-9.1463, 29.8553)
  line L236 (-9.1463, 29.8553) -> (-8.5896, 30.0202)
  line L237 (-8.5896, 30.0202) -> (-8.2981, 29.6783)
  line L238 (-8.2981, 29.6783) -> (-8.0228, 29.3309)
  line L239 (-8.0228, 29.3309) -> (-7.7646, 28.9778)
  line L240 (-7.7646, 28.9778) -> (-7.5249, 28.619)
  line L241 (-7.5249, 28.619) -> (-7.3057, 28.2542)
  line L242 (-7.3057, 28.2542) -> (-7.2047, 28.0694)
  line L243 (-7.2047, 28.0694) -> (-7.1566, 27.9763)
  line L244 (-7.1566, 27.9763) -> (-7.1102, 27.8828)
  line L245 (-7.1102, 27.8828) -> (-6.3233, 28.0717)
  line L246 (-6.3233, 28.0717) -> (-6.3244, 28.1761)
  line L247 (-6.3244, 28.1761) -> (-6.3238, 28.2808)
  line L248 (-6.3238, 28.2808) -> (-6.3177, 28.4913)
  line L249 (-6.3177, 28.4913) -> (-6.288, 28.9159)
  line L250 (-6.288, 28.9159) -> (-6.2373, 29.3444)
  line L251 (-6.2373, 29.3444) -> (-6.1676, 29.7763)
  line L252 (-6.1676, 29.7763) -> (-6.08, 30.2109)
  line L253 (-6.08, 30.2109) -> (-5.9755, 30.6478)
  line L254 (-5.9755, 30.6478) -> (-5.4046, 30.7536)
  line L255 (-5.4046, 30.7536) -> (-5.1504, 30.3832)
  line L256 (-5.1504, 30.3832) -> (-4.9129, 30.0088)
  line L257 (-4.9129, 30.0088) -> (-4.693, 29.6306)
  line L258 (-4.693, 29.6306) -> (-4.4922, 29.2487)
  line L259 (-4.4922, 29.2487) -> (-4.3123, 28.863)
  line L260 (-4.3123, 28.863) -> (-4.2312, 28.6687)
  line L261 (-4.2312, 28.6687) -> (-4.1931, 28.5711)
  line L262 (-4.1931, 28.5711) -> (-4.1567, 28.4733)
  line L263 (-4.1567, 28.4733) -> (-3.3543, 28.5789)
  line L264 (-3.3543, 28.5789) -> (-3.3446, 28.6828)
  line L265 (-3.3446, 28.6828) -> (-3.333, 28.7869)
  line L266 (-3.333, 28.7869) -> (-3.305, 28.9957)
  line L267 (-3.305, 28.9957) -> (-3.231, 29.4148)
  line L268 (-3.231, 29.4148) -> (-3.1359, 29.8357)
  line L269 (-3.1359, 29.8357) -> (-3.0213, 30.2578)
  line L270 (-3.0213, 30.2578) -> (-2.8888, 30.6809)
  line L271 (-2.8888, 30.6809) -> (-2.7392, 31.1045)
  line L272 (-2.7392, 31.1045) -> (-2.1604, 31.1501)
  line L273 (-2.1604, 31.1501) -> (-1.9463, 30.7551)
  line L274 (-1.9463, 30.7551) -> (-1.7492, 30.358)
  line L275 (-1.7492, 30.358) -> (-1.5701, 29.9589)
  line L276 (-1.5701, 29.9589) -> (-1.4102, 29.5581)
  line L277 (-1.4102, 29.5581) -> (-1.2716, 29.1557)
  line L278 (-1.2716, 29.1557) -> (-1.2113, 28.9539)
  line L279 (-1.2113, 28.9539) -> (-1.1836, 28.8529)
  line L280 (-1.1836, 28.8529) -> (-1.1577, 28.7518)
  line L281 (-1.1577, 28.7518) -> (-0.3487, 28.773)
  line L282 (-0.3487, 28.773) -> (-0.3281, 28.8753)
  line L283 (-0.3281, 28.8753) -> (-0.3057, 28.9776)
  line L284 (-0.3057, 28.9776) -> (-0.256, 29.1823)
  line L285 (-0.256, 29.1823) -> (-0.1387, 29.5914)
  line L286 (-0.1387, 29.5914) -> (0, 30)
  line L287 (0, 30) -> (0.158, 30.4079)
  line L288 (0.158, 30.4079) -> (0.3341, 30.8148)
  line L289 (0.3341, 30.8148) -> (0.5271, 31.2205)
  line L290 (0.5271, 31.2205) -> (1.1075, 31.2053)
  line L291 (1.1075, 31.2053) -> (1.2791, 30.7901)
  line L292 (1.2791, 30.7901) -> (1.4336, 30.3745)
  line L293 (1.4336, 30.3745) -> (1.5701, 29.9589)
  line L294 (1.5701, 29.9589) -> (1.6872, 29.5436)
  line L295 (1.6872, 29.5436) -> (1.7829, 29.1289)
  line L296 (1.7829, 29.1289) -> (1.8218, 28.9219)
  line L297 (1.8218, 28.9219) -> (1.8388, 28.8186)
  line L298 (1.8388, 28.8186) -> (1.854, 28.7153)
  line L299 (1.854, 28.7153) -> (2.6608, 28.6518)
  line L300 (2.6608, 28.6518) -> (2.692, 28.7514)
  line L301 (2.692, 28.7514) -> (2.725, 28.8508)
  line L302 (2.725, 28.8508) -> (2.7958, 29.0492)
  line L303 (2.7958, 29.0492) -> (2.9552, 29.4438)
  line L304 (2.9552, 29.4438) -> (3.1359, 29.8357)
  line L305 (3.1359, 29.8357) -> (3.3356, 30.2248)
  line L306 (3.3356, 30.2248) -> (3.5533, 30.6111)
  line L307 (3.5533, 30.6111) -> (3.7877, 30.9943)
  line L308 (3.7877, 30.9943) -> (4.3633, 30.9185)
  line L309 (4.3633, 30.9185) -> (4.4905, 30.4877)
  line L310 (4.4905, 30.4877) -> (4.6008, 30.0582)
  line L311 (4.6008, 30.0582) -> (4.693, 29.6307)
  line L312 (4.693, 29.6307) -> (4.7661, 29.2054)
  line L313 (4.7661, 29.2054) -> (4.8179, 28.783)
  line L314 (4.8179, 28.783) -> (4.835, 28.5731)
  line L315 (4.835, 28.5731) -> (4.8411, 28.4685)
  line L316 (4.8411, 28.4685) -> (4.8454, 28.3642)
  line L317 (4.8454, 28.3642) -> (5.6412, 28.2167)
  line L318 (5.6412, 28.2167) -> (5.6826, 28.3125)
  line L319 (5.6826, 28.3125) -> (5.7258, 28.408)
  line L320 (5.7258, 28.408) -> (5.817, 28.5978)
  line L321 (5.817, 28.5978) -> (6.0168, 28.9736)
  line L322 (6.0168, 28.9736) -> (6.2373, 29.3444)
  line L323 (6.2373, 29.3444) -> (6.4767, 29.7106)
  line L324 (6.4767, 29.7106) -> (6.7335, 30.072)
  line L325 (6.7335, 30.072) -> (7.0067, 30.4286)
  line L326 (7.0067, 30.4286) -> (7.5713, 30.2931)
  line L327 (7.5713, 30.2931) -> (7.6528, 29.8513)
  line L328 (7.6528, 29.8513) -> (7.7175, 29.4127)
  line L329 (7.7175, 29.4127) -> (7.7646, 28.9778)
  line L330 (7.7646, 28.9778) -> (7.7928, 28.5472)
  line L331 (7.7928, 28.5472) -> (7.8002, 28.1217)
  line L332 (7.8002, 28.1217) -> (7.7952, 27.9111)
  line L333 (7.7952, 27.9111) -> (7.7904, 27.8065)
  line L334 (7.7904, 27.8065) -> (7.7838, 27.7023)
  line L335 (7.7838, 27.7023) -> (8.5597, 27.4725)
  line L336 (8.5597, 27.4725) -> (8.6109, 27.5634)
  line L337 (8.6109, 27.5634) -> (8.6638, 27.6538)
  line L338 (8.6638, 27.6538) -> (8.7744, 27.8331)
  line L339 (8.7744, 27.8331) -> (9.0124, 28.1859)
  line L340 (9.0124, 28.1859) -> (9.2705, 28.5317)
  line L341 (9.2705, 28.5317) -> (9.5468, 28.8708)
  line L342 (9.5468, 28.8708) -> (9.84, 29.2034)
  line L343 (9.84, 29.2034) -> (10.149, 29.5295)
  line L344 (10.149, 29.5295) -> (10.6963, 29.3357)
  line L345 (10.6963, 29.3357) -> (10.7312, 28.8878)
  line L346 (10.7312, 28.8878) -> (10.7497, 28.4449)
  line L347 (10.7497, 28.4449) -> (10.751, 28.0074)
  line L348 (10.751, 28.0074) -> (10.734, 27.5762)
  line L349 (10.734, 27.5762) -> (10.697, 27.1523)
  line L350 (10.697, 27.1523) -> (10.67, 26.9434)
  line L351 (10.67, 26.9434) -> (10.6543, 26.8398)
  line L352 (10.6543, 26.8398) -> (10.6368, 26.737)
  line L353 (10.6368, 26.737) -> (11.3845, 26.4272)
  line L354 (11.3845, 26.4272) -> (11.4449, 26.5123)
  line L355 (11.4449, 26.5123) -> (11.507, 26.5967)
  line L356 (11.507, 26.5967) -> (11.6356, 26.7635)
  line L357 (11.6356, 26.7635) -> (11.9092, 27.0895)
  line L358 (11.9092, 27.0895) -> (12.2021, 27.4064)
  line L359 (12.2021, 27.4064) -> (12.5124, 27.7147)
  line L360 (12.5124, 27.7147) -> (12.8387, 28.0148)
  line L361 (12.8387, 28.0148) -> (13.1801, 28.3069)
  line L362 (13.1801, 28.3069) -> (13.7041, 28.057)
  line L363 (13.7041, 28.057) -> (13.692, 27.6079)
  line L364 (13.692, 27.6079) -> (13.6641, 27.1654)
  line L365 (13.6641, 27.1654) -> (13.6197, 26.7302)
  line L366 (13.6197, 26.7302) -> (13.5577, 26.3032)
  line L367 (13.5577, 26.3032) -> (13.4766, 25.8854)
  line L368 (13.4766, 25.8854) -> (13.4279, 25.6805)
  line L369 (13.4279, 25.6805) -> (13.4014, 25.5791)
  line L370 (13.4014, 25.5791) -> (13.3733, 25.4786)
  line L371 (13.3733, 25.4786) -> (14.0845, 25.0925)
  line L372 (14.0845, 25.0925) -> (14.1535, 25.1708)
  line L373 (14.1535, 25.1708) -> (14.2241, 25.2482)
  line L374 (14.2241, 25.2482) -> (14.3695, 25.4006)
  line L375 (14.3695, 25.4006) -> (14.6756, 25.6962)
  line L376 (14.6756, 25.6962) -> (15, 25.9808)
  line L377 (15, 25.9808) -> (15.3408, 26.255)
  line L378 (15.3408, 26.255) -> (15.6967, 26.5194)
  line L379 (15.6967, 26.5194) -> (16.0667, 26.7741)
  line L380 (16.0667, 26.7741) -> (16.5618, 26.4708)
  line L381 (16.5618, 26.4708) -> (16.5028, 26.0254)
  line L382 (16.5028, 26.0254) -> (16.4288, 25.5883)
  line L383 (16.4288, 25.5883) -> (16.3392, 25.1601)
  line L384 (16.3392, 25.1601) -> (16.2329, 24.7419)
  line L385 (16.2329, 24.7419) -> (16.1085, 24.3349)
  line L386 (16.1085, 24.3349) -> (16.0387, 24.1362)
  line L387 (16.0387, 24.1362) -> (16.0018, 24.0382)
  line L388 (16.0018, 24.0382) -> (15.9633, 23.9412)
  line L389 (15.9633, 23.9412) -> (16.6303, 23.4828)
  line L390 (16.6303, 23.4828) -> (16.7071, 23.5535)
  line L391 (16.7071, 23.5535) -> (16.7853, 23.6231)
  line L392 (16.7853, 23.6231) -> (16.9458, 23.7594)
  line L393 (16.9458, 23.7594) -> (17.2812, 24.0214)
  line L394 (17.2812, 24.0214) -> (17.6336, 24.2705)
  line L395 (17.6336, 24.2705) -> (18.0012, 24.5076)
  line L396 (18.0012, 24.5076) -> (18.3827, 24.7333)
  line L397 (18.3827, 24.7333) -> (18.7774, 24.948)
  line L398 (18.7774, 24.948) -> (19.238, 24.5946)
  line L399 (19.238, 24.5946) -> (19.1328, 24.1578)
  line L400 (19.1328, 24.1578) -> (19.0135, 23.7308)
  line L401 (19.0135, 23.7308) -> (18.8796, 23.3144)
  line L402 (18.8796, 23.3144) -> (18.7302, 22.9096)
  line L403 (18.7302, 22.9096) -> (18.5639, 22.5178)
  line L404 (18.5639, 22.5178) -> (18.4738, 22.3275)
  line L405 (18.4738, 22.3275) -> (18.4268, 22.2339)
  line L406 (18.4268, 22.2339) -> (18.3784, 22.1414)
  line L407 (18.3784, 22.1414) -> (18.9938, 21.6158)
  line L408 (18.9938, 21.6158) -> (19.0776, 21.6781)
  line L409 (19.0776, 21.6781) -> (19.1626, 21.7391)
  line L410 (19.1626, 21.7391) -> (19.3365, 21.8579)
  line L411 (19.3365, 21.8579) -> (19.6974, 22.0835)
  line L412 (19.6974, 22.0835) -> (20.0739, 22.2943)
  line L413 (20.0739, 22.2943) -> (20.4643, 22.4917)
  line L414 (20.4643, 22.4917) -> (20.8674, 22.6763)
  line L415 (20.8674, 22.6763) -> (21.2823, 22.8486)
  line L416 (21.2823, 22.8486) -> (21.7035, 22.4489)
  line L417 (21.7035, 22.4489) -> (21.5531, 22.0256)
  line L418 (21.5531, 22.0256) -> (21.3899, 21.6134)
  line L419 (21.3899, 21.6134) -> (21.2132, 21.2132)
  line L420 (21.2132, 21.2132) -> (21.0223, 20.8262)
  line L421 (21.0223, 20.8262) -> (20.816, 20.454)
  line L422 (20.816, 20.454) -> (20.7064, 20.2741)
  line L423 (20.7064, 20.2741) -> (20.6499, 20.1859)
  line L424 (20.6499, 20.1859) -> (20.5921, 20.099)
  line L425 (20.5921, 20.099) -> (21.1492, 19.512)
  line L426 (21.1492, 19.512) -> (21.239, 19.5652)
  line L427 (21.239, 19.5652) -> (21.33, 19.617)
  line L428 (21.33, 19.617) -> (21.5154, 19.717)
  line L429 (21.5154, 19.717) -> (21.8979, 19.9035)
  line L430 (21.8979, 19.9035) -> (22.2943, 20.0739)
  line L431 (22.2943, 20.0739) -> (22.7032, 20.2294)
  line L432 (22.7032, 20.2294) -> (23.1234, 20.3709)
  line L433 (23.1234, 20.3709) -> (23.5541, 20.4988)
  line L434 (23.5541, 20.4988) -> (23.9311, 20.0573)
  line L435 (23.9311, 20.0573) -> (23.7374, 19.652)
  line L436 (23.7374, 19.652) -> (23.5319, 19.2591)
  line L437 (23.5319, 19.2591) -> (23.3144, 18.8796)
  line L438 (23.3144, 18.8796) -> (23.0841, 18.5147)
  line L439 (23.0841, 18.5147) -> (22.84, 18.1661)
  line L440 (22.84, 18.1661) -> (22.7122, 17.9986)
  line L441 (22.7122, 17.9986) -> (22.6468, 17.9169)
  line L442 (22.6468, 17.9169) -> (22.5802, 17.8365)
  line L443 (22.5802, 17.8365) -> (23.0729, 17.1944)
  line L444 (23.0729, 17.1944) -> (23.1678, 17.2379)
  line L445 (23.1678, 17.2379) -> (23.2637, 17.2799)
  line L446 (23.2637, 17.2799) -> (23.4585, 17.36)
  line L447 (23.4585, 17.36) -> (23.8584, 17.5056)
  line L448 (23.8584, 17.5056) -> (24.2705, 17.6336)
  line L449 (24.2705, 17.6336) -> (24.6934, 17.7455)
  line L450 (24.6934, 17.7455) -> (25.1261, 17.8422)
  line L451 (25.1261, 17.8422) -> (25.5677, 17.9245)
  line L452 (25.5677, 17.9245) -> (25.8966, 17.446)
  line L453 (25.8966, 17.446) -> (25.6615, 17.0631)
  line L454 (25.6615, 17.0631) -> (25.4161, 16.6939)
  line L455 (25.4161, 16.6939) -> (25.1601, 16.3392)
  line L456 (25.1601, 16.3392) -> (24.8929, 16.0003)
  line L457 (24.8929, 16.0003) -> (24.6137, 15.6791)
  line L458 (24.6137, 15.6791) -> (24.4692, 15.526)
  line L459 (24.4692, 15.526) -> (24.3955, 15.4515)
  line L460 (24.3955, 15.4515) -> (24.3209, 15.3785)
  line L461 (24.3209, 15.3785) -> (24.7438, 14.6884)
  line L462 (24.7438, 14.6884) -> (24.8427, 14.7218)
  line L463 (24.8427, 14.7218) -> (24.9425, 14.7536)
  line L464 (24.9425, 14.7536) -> (25.1446, 14.8128)
  line L465 (25.1446, 14.8128) -> (25.5575, 14.9158)
  line L466 (25.5575, 14.9158) -> (25.9808, 15)
  line L467 (25.9808, 15) -> (26.413, 15.0671)
  line L468 (26.413, 15.0671) -> (26.8534, 15.1181)
  line L469 (26.8534, 15.1181) -> (27.3013, 15.1537)
  line L470 (27.3013, 15.1537) -> (27.5783, 14.6435)
  line L471 (27.5783, 14.6435) -> (27.3045, 14.2873)
  line L472 (27.3045, 14.2873) -> (27.0219, 13.9457)
  line L473 (27.0219, 13.9457) -> (26.7302, 13.6197)
  line L474 (26.7302, 13.6197) -> (26.4291, 13.3107)
  line L475 (26.4291, 13.3107) -> (26.1178, 13.0204)
  line L476 (26.1178, 13.0204) -> (25.958, 12.8832)
  line L477 (25.958, 12.8832) -> (25.877, 12.8168)
  line L478 (25.877, 12.8168) -> (25.7952, 12.752)
  line L479 (25.7952, 12.752) -> (26.1436, 12.0215)
  line L480 (26.1436, 12.0215) -> (26.2455, 12.0443)
  line L481 (26.2455, 12.0443) -> (26.348, 12.0655)
  line L482 (26.348, 12.0655) -> (26.5552, 12.1033)
  line L483 (26.5552, 12.1033) -> (26.9767, 12.1626)
  line L484 (26.9767, 12.1626) -> (27.4064, 12.2021)
  line L485 (27.4064, 12.2021) -> (27.8433, 12.2236)
  line L486 (27.8433, 12.2236) -> (28.2866, 12.2283)
  line L487 (28.2866, 12.2283) -> (28.7357, 12.2169)
  line L488 (28.7357, 12.2169) -> (28.9579, 11.6805)
  line L489 (28.9579, 11.6805) -> (28.6484, 11.3549)
  line L490 (28.6484, 11.3549) -> (28.3316, 11.0447)
  line L491 (28.3316, 11.0447) -> (28.0074, 10.751)
  line L492 (28.0074, 10.751) -> (27.6756, 10.4752)
  line L493 (27.6756, 10.4752) -> (27.3357, 10.219)
  line L494 (27.3357, 10.219) -> (27.1625, 10.0993)
  line L495 (27.1625, 10.0993) -> (27.075, 10.0417)
  line L496 (27.075, 10.0417) -> (26.9868, 9.9858)
  line L497 (26.9868, 9.9858) -> (27.257, 9.2229)
  line L498 (27.257, 9.2229) -> (27.3607, 9.235)
  line L499 (27.3607, 9.235) -> (27.4649, 9.2453)
  line L500 (27.4649, 9.2453) -> (27.6749, 9.2613)
  line L501 (27.6749, 9.2613) -> (28.1002, 9.2761)
  line L502 (28.1002, 9.2761) -> (28.5317, 9.2705)
  line L503 (28.5317, 9.2705) -> (28.9685, 9.2463)
  line L504 (28.9685, 9.2463) -> (29.4098, 9.2046)
  line L505 (29.4098, 9.2046) -> (29.8553, 9.1463)
  line L506 (29.8553, 9.1463) -> (30.0202, 8.5896)
  line L507 (30.0202, 8.5896) -> (29.6783, 8.2981)
  line L508 (29.6783, 8.2981) -> (29.3309, 8.0228)
  line L509 (29.3309, 8.0228) -> (28.9778, 7.7646)
  line L510 (28.9778, 7.7646) -> (28.619, 7.5249)
  line L511 (28.619, 7.5249) -> (28.2542, 7.3057)
  line L512 (28.2542, 7.3057) -> (28.0694, 7.2047)
  line L513 (28.0694, 7.2047) -> (27.9763, 7.1566)
  line L514 (27.9763, 7.1566) -> (27.8828, 7.1102)
  line L515 (27.8828, 7.1102) -> (28.0717, 6.3233)
  line L516 (28.0717, 6.3233) -> (28.1761, 6.3244)
  line L517 (28.1761, 6.3244) -> (28.2808, 6.3238)
  line L518 (28.2808, 6.3238) -> (28.4913, 6.3177)
  line L519 (28.4913, 6.3177) -> (28.9159, 6.288)
  line L520 (28.9159, 6.288) -> (29.3444, 6.2374)
  line L521 (29.3444, 6.2374) -> (29.7763, 6.1676)
  line L522 (29.7763, 6.1676) -> (30.2109, 6.08)
  line L523 (30.2109, 6.08) -> (30.6478, 5.9755)
  line L524 (30.6478, 5.9755) -> (30.7536, 5.4046)
  line L525 (30.7536, 5.4046) -> (30.3832, 5.1505)
  line L526 (30.3832, 5.1505) -> (30.0088, 4.9129)
  line L527 (30.0088, 4.9129) -> (29.6306, 4.693)
  line L528 (29.6306, 4.693) -> (29.2487, 4.4922)
  line L529 (29.2487, 4.4922) -> (28.863, 4.3123)
  line L530 (28.863, 4.3123) -> (28.6687, 4.2312)
  line L531 (28.6687, 4.2312) -> (28.5711, 4.1931)
  line L532 (28.5711, 4.1931) -> (28.4733, 4.1567)
  line L533 (28.4733, 4.1567) -> (28.5789, 3.3543)
  line L534 (28.5789, 3.3543) -> (28.6828, 3.3446)
  line L535 (28.6828, 3.3446) -> (28.7869, 3.333)
  line L536 (28.7869, 3.333) -> (28.9957, 3.305)
  line L537 (28.9957, 3.305) -> (29.4148, 3.231)
  line L538 (29.4148, 3.231) -> (29.8357, 3.1359)
  line L539 (29.8357, 3.1359) -> (30.2578, 3.0213)
  line L540 (30.2578, 3.0213) -> (30.6809, 2.8888)